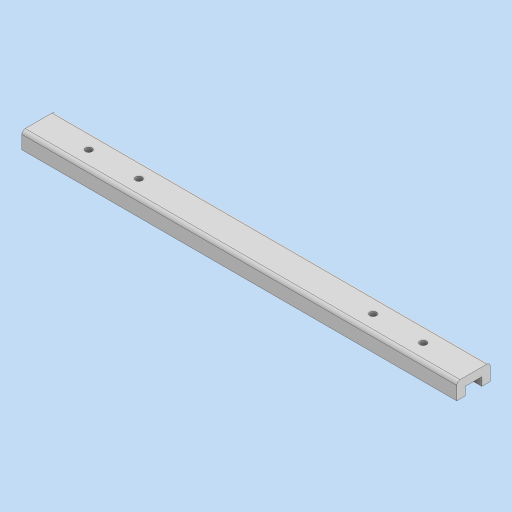
# Autodesk Inventor part: BASE_DE_PRUEBA
Saved by Autodesk Inventor 2024 (Build 280153000, 153)
## iProperties
Created: 2024-10-01
Part Number: BASE_DE_PRUEBA
Material: Generic
Document SubType Name: Modeling
Designer: MxMon
Density: 1 g/cm^3
Appearance: Default
Author: MxMon
Autodesk Inventor part; units mm, degrees
ref_plane "YZ Plane" through (0, 0, 0) normal (1, 0, 0) x (0, 1, 0)
ref_plane "XZ Plane" through (0, 0, 0) normal (0, 1, 0) x (-1, 0, 0)
ref_plane "XY Plane" through (0, 0, 0) normal (0, 0, 1) x (1, 0, 0)
sketch "Sketch2" plane through (0, 0, 0) normal (0, 1, 0) x (-1, 0, 0)
  line L0 (130, 10) -> (-130, 10)
  line L1 (-130, 10) -> (-130, -10)
  line L2 (-130, -10) -> (130, -10)
  line L3 (130, -10) -> (130, 10)
  line L4 (130, 10) -> (-130, -10) construction
  line L5 (-130, 10) -> (130, -10) construction
  point P0 (0, 0)
  dimension "d6" = 260
  dimension "d7" = 20
  constraints: 12 end point, 2 midpoint, 2 parallel, 1 horizontal, 1 perpendicular
  measures "d6" distance of L2.end L1.end
  measures "d7" distance of L1.end L0.end
extrude "Extrusion2" add sketch "Sketch2" along normal blind 5
sketch "Sketch3" plane through (0, 0, 0) normal (0, -1, 0) x (1, 0, 0)
  line L0 (-130, -10) -> (-130, 10) projected
  line L1 (-130, 10) -> (130, 10)
  line L2 (130, 10) -> (130, 5)
  line L3 (130, 5) -> (-130, 5)
  line L4 (-130, 5) -> (-130, 10)
  line L5 (130, -10) -> (-130, -10) projected
  line L6 (130, -10) -> (-130, -10)
  line L7 (-130, -10) -> (-130, -5)
  line L8 (-130, -5) -> (130, -5)
  line L9 (130, -5) -> (130, -10)
  point P0 (0, 0)
  dimension "d10" = 260
  dimension "d11" = 5
  dimension "d13" = 5
  constraints: 16 end point, 4 parallel, 2 horizontal, 2 perpendicular, 1 point on line
  measures "d10" distance of L2.end L3.end
  measures "d11" distance of L1.end L2.end
  measures "d13" distance of L0.start L7.end
extrude "Extrusion3" add sketch "Sketch3" along normal blind 5
fillet "Fillet1" radius 2 2 edges at (0, 5, 10) (0, 5, -10)
sketch "Sketch5" plane through (0, 5, 0) normal (0, 1, 0) x (1, 0, 0)
  point P0 (0, 0)
  point P1 (100, 0)
  point P2 (70, 0)
  point P3 (-70, 0)
  point P4 (-100, 0)
  dimension "d31" = 70
  dimension "d32" = 70
  dimension "d33" = 30
  dimension "d34" = 30
  constraints: 4 horizontal alignment
  measures "d31" distance of point (0, 0) point (70, 0)
  measures "d32" distance of point (-70, 0) point (0, 0)
  measures "d33" distance of point (-100, 0) point (-70, 0)
  measures "d34" distance of point (70, 0) point (100, 0)
hole "Hole2" at (100, 5, 0) at (70, 5, 0) at (-70, 5, 0) at (-100, 5, 0) direction (0, -1, 0) diameter 4 end through all
body "Solid2"
